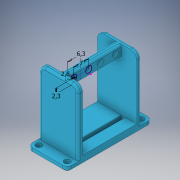
# Autodesk Inventor part: Stewart-KST215-Servo-Holder
Saved by Autodesk Inventor 2018.2 (Build 222227000, 227)
## iProperties
Created: 2018-02-17
Part Number: Stewart-KST215-Servo-Holder
Material: Generisch
Document SubType Name: Modeling
Designer: JochenAlt
Density: 1 g/cm^3
Appearance: Vorgabe
Author: JochenAlt
Autodesk Inventor part; units mm, degrees
ref_plane "YZ Plane" through (0, 0, 0) normal (1, 0, 0) x (0, 1, 0)
ref_plane "XZ Plane" through (0, 0, 0) normal (0, 1, 0) x (-1, 0, 0)
ref_plane "XY Plane" through (0, 0, 0) normal (0, 0, 1) x (1, 0, 0)
sketch "Skizze1" plane through (0, 0, 0) normal (0, 0, 1) x (1, 0, 0)
  line L0 (0, 27.8099) -> (0, -27.8099) construction
  line L1 (-8.901, 0) -> (53.4059, 0) construction
  line L2 (17.4907, 0.15) -> (44.0907, 0.15) construction
  line L3 (44.0907, 0.15) -> (44.0907, 12.15) construction
  line L4 (44.0907, 12.15) -> (17.4907, 12.15) construction
  line L5 (17.4907, 12.15) -> (17.4907, 0.15) construction
  line L6 (17.4907, -0.15) -> (44.0907, -0.15) construction
  line L7 (44.0907, -0.15) -> (44.0907, -12.15) construction
  line L8 (44.0907, -12.15) -> (17.4907, -12.15) construction
  line L9 (17.4907, -12.15) -> (17.4907, -0.15) construction
  line L10 (38.5907, 12.15) -> (38.5907, 0.15) construction
  line L11 (37.3907, 12.15) -> (37.3907, 0.15) construction
  line L12 (37.3907, -0.15) -> (37.3907, -12.15) construction
  line L13 (38.5907, -12.15) -> (38.5907, -0.15) construction
  line L14 (44.0907, 2) -> (44.0907, 12.45)
  line L15 (44.0907, 12.45) -> (26.0907, 12.45)
  line L16 (26.0907, -12.45) -> (44.0907, -12.45)
  line L17 (44.0907, -12.45) -> (44.0907, 2)
  line L18 (26.0907, 12.45) -> (26.0907, 17.45)
  line L19 (28.0907, 19.45) -> (42.0907, 19.45)
  line L20 (44.0907, 17.45) -> (44.0907, 12.45)
  line L21 (26.0907, -12.45) -> (26.0907, -17.45)
  line L22 (28.0907, -19.45) -> (42.0907, -19.45)
  line L23 (44.0907, -12.45) -> (44.0907, -17.45)
  circle A0 centre (41.5907, 16.95) radius 1.35
  circle A1 centre (28.5907, 16.95) radius 1.35
  circle A2 centre (28.5907, -16.95) radius 1.35
  circle A3 centre (41.5907, -16.95) radius 1.35
  line L24 (28.5907, 16.95) -> (41.5907, 16.95) construction
  arc A4 (28.0907, 19.45) -> (26.0907, 17.45) centre (28.0907, 17.45) ccw
  arc A5 (44.0907, 17.45) -> (42.0907, 19.45) centre (42.0907, 17.45) ccw
  line L25 (28.0907, 17.45) -> (42.0907, 17.45) construction
  arc A6 (26.0907, -17.45) -> (28.0907, -19.45) centre (28.0907, -17.45) ccw
  arc A7 (42.0907, -19.45) -> (44.0907, -17.45) centre (42.0907, -17.45) ccw
  line L26 (38.8907, 12.45) -> (38.8907, 0.15)
  line L27 (37.0907, 12.45) -> (37.0907, 0.15)
  line L28 (37.0907, 0.15) -> (37.0907, -12.45)
  line L29 (38.8907, -12.45) -> (38.8907, 0.15)
  line L30 (26.0907, 14.45) -> (44.0907, 14.45)
  line L31 (35.0907, 19.45) -> (35.0907, 14.45) construction
  line L32 (26.0907, -14.45) -> (44.0907, -14.45)
  line L33 (35.0907, 14.45) -> (35.0907, 19.45) construction
  line L34 (34.0907, -12.45) -> (34.0907, 12.45)
  line L35 (26.0907, -12.45) -> (26.0907, 12.45)
  point P0 (0, 0)
  dimension "d59" = 12
  dimension "d62" = 1.2
  dimension "d64" = 0.3
  dimension "d69" = 2.7
  dimension "d70" = 13
  dimension "d71" = 7
  dimension "d72" = 4
  dimension "d74" = 0.3
  dimension "d75" = 0.3
  dimension "d77" = 2
  dimension "d98" = 26.6
  dimension "d99" = 0.3
  dimension "d100" = 3
  dimension "d101" = 5.5
  constraints: 68 end point, 19 point on line, 12 perpendicular, 10 parallel, 8 centre point, 8 point on circle, 8 symmetric about line, 8 tangent, 6 equal radius, 4 midpoint, 2 collinear, 2 equal length, 1 coincident, 1 vertical, 5 other
  measures "d59" distance between parallel lines of L2 L4
  measures "d62" distance between parallel lines of L10 L11
  measures "d64" distance between parallel lines of L4 L15
  measures "d69" diameter of A0
  measures "d70" distance of L24.end L24.start
  measures "d71" distance between parallel lines of L15 L19
  measures "d72" diameter of A4
  measures "d74" distance between parallel lines of L10 L26
  measures "d75" distance between parallel lines of L11 L27
  measures "d77" distance between parallel lines of L15 L30
  measures "d98" distance between parallel lines of L17 L9
  measures "d99" distance between parallel lines of L2 L6
  measures "d100" distance between parallel lines of L34 L28
  measures "d101" distance between parallel lines of L3 L10
extrude "Extrusion1" add sketch "Skizze1" along normal blind 2 contours L17 L16 L29 L26 L15 L14 | L15 L18 L30 L20 | L23 L32 L21 L16 | L30 L18 A4 L19 A5 L20 | L23 A7 L22 A6 L21 L32 | L27 L28 L16 L34 L15 | L34 L16 L35 L15
extrude "Extrusion2" add sketch "Skizze1" along normal blind 3.5 contours L17 L16 L29 L26 L15 L14 | L15 L18 L30 L20 | L23 L32 L21 L16 | L27 L28 L16 L34 L15 | L34 L16 L35 L15
extrude "Extrusion4" add sketch "Skizze1" along normal blind 27 contours L15 L18 L30 L20 | L23 L32 L21 L16
extrude "Extrusion5" add sketch "Skizze1" along normal blind 4.7 from surface at 27 contours L15 L18 L30 L20 | L23 L32 L21 L16 | L27 L28 L16 L34 L15
sketch "Skizze4" plane through (37.0907, -14.3441, 31.7) normal (1, 0, 0) x (0, 0, -1)
  circle A0 centre (2.4, 4.6941) radius 1.4
  circle A1 centre (2.4, 11.6941) radius 1.4
  line L0 (4.7, 12.6) -> (4.7, 3.7882) construction
  line L1 (2.4, 4.6941) -> (2.4, 11.6941) construction
  line L2 (4.7, 12.6) -> (4.7, 3.7882) construction
  line L3 (4.7, 8.1941) -> (0, 8.1941) construction
  line L4 (28.2, 1.8941) -> (0, 1.8941) projected
  point P0 (31.7, 14.3441)
  point P1 (31.7, 1.8941)
  dimension "d80" = 2.8
  dimension "d81" = 2.3
  dimension "d82" = 7
  dimension "d102" = 6.3
  constraints: 4 end point, 2 centre point, 1 equal radius, 1 midpoint, 1 parallel, 1 symmetric about line
  measures "d80" diameter of A0
  measures "d81" distance between parallel lines of L0 L1
  measures "d82" distance of L1.end L1.start
  measures "d102" distance between parallel lines of L3 L4
extrude "Extrusion9" cut sketch "Skizze4" against normal up to next
sketch "Skizze5" plane through (37.0907, 1.8131, 31.7) normal (1, 0, 0) x (0, 0, -1)
  circle A0 centre (2.4, 0.8369) radius 1.4
  circle A1 centre (2.4, 7.8369) radius 1.4
  line L0 (2.4, 0.8369) -> (2.4, 7.8369) construction
  line L1 (0, 12.6) -> (4.7, 12.6) construction
  line L2 (0, 4.3369) -> (4.7, 4.3369) construction
  line L3 (28.2, 10.6369) -> (0, 10.6369) projected
  point P0 (31.7, -1.8131)
  point P1 (4.7, 8.6738)
  point P2 (31.7, 10.6369)
  dimension "d85" = 7
  dimension "d87" = 2.8
  dimension "d103" = 6.3
  constraints: 4 end point, 2 centre point, 1 equal radius, 1 symmetric about line, 1 vertical
  measures "d85" distance of L0.end L0.start
  measures "d87" diameter of A0
  measures "d103" distance between parallel lines of L2 L3
extrude "Extrusion10" cut sketch "Skizze5" against normal up to next
fillet "Rundung4" radius 3 4 edges at (44.0907, 13.45, 31.7) (44.0907, -13.45, 31.7) (26.0907, -13.45, 31.7) (26.0907, 13.45, 31.7)
fillet "Rundung4" radius 1 8 edges at (35.0907, -14.45, 31.7) (44.0907, -14.45, 16.85) (35.0907, 14.45, 31.7) (44.0907, 14.45, 16.85) (37.0907, 0, 31.7) (34.0907, 0, 31.7) (26.0907, 14.45, 16.85) (26.0907, -14.45, 16.85)
chamfer "Fase3" distance 0.5 angle 45 7 edges at (26.6765, 18.8642, 0) (35.0907, 19.45, 0) (43.5049, 18.8642, 0) (44.0907, 0, 0) (26.6765, -18.8642, 0) (35.0907, -19.45, 0) (43.5049, -18.8642, 0)
